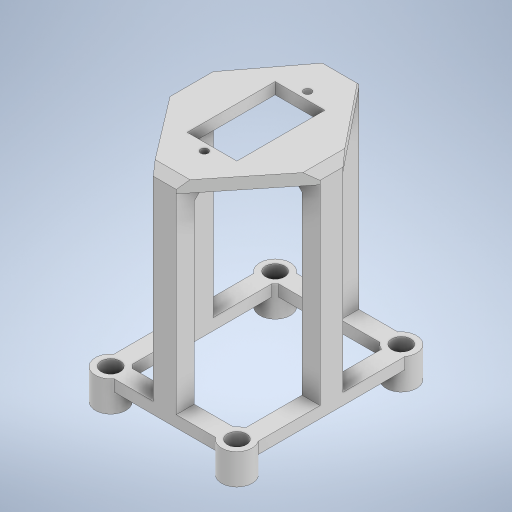
# Autodesk Inventor part: ServoMount
Saved by Autodesk Inventor 2024.2 (Build 282272000, 272)
## iProperties
Created: 2024-04-02
Part Number: ServoMount
Material: Generic
Document SubType Name: Modeling
Designer: ringl
Density: 1 g/cm^3
Appearance: Default
Author: ringl
Autodesk Inventor part; units mm, degrees
ref_plane "YZ Plane" through (0, 0, 0) normal (1, 0, 0) x (0, 1, 0)
ref_plane "XZ Plane" through (0, 0, 0) normal (0, 1, 0) x (-1, 0, 0)
ref_plane "XY Plane" through (0, 0, 0) normal (0, 0, 1) x (1, 0, 0)
sketch "Sketch1" plane through (0, 0, 0) normal (0, 1, 0) x (-1, 0, 0)
  circle A0 centre (0, 0) radius 2.5
  circle A1 centre (0, -43) radius 2.5
  circle A2 centre (-33, 0) radius 2.5
  circle A3 centre (-33, -43) radius 2.5
  line L0 (-3.2369, 2.35) -> (-29.7631, 2.35)
  line L1 (-29.7631, -2.35) -> (-3.2369, -2.35)
  line L2 (-2.35, -3.2369) -> (-2.35, -39.7631)
  line L3 (-3.2369, -40.65) -> (-29.7631, -40.65)
  line L4 (-31.5369, -39.2772) -> (-31.5369, -3.7228)
  line L5 (-36.2369, -2.35) -> (-36.2369, -40.65)
  line L6 (-3.2369, -45.35) -> (-29.7631, -45.35)
  arc A4 (-29.7631, -40.65) -> (-31.5369, -39.2772) centre (-33, -43) ccw
  arc A5 (-36.2369, -40.65) -> (-29.7631, -45.35) centre (-33, -43) ccw
  line L7 (2.35, -3.2369) -> (2.35, -39.7631)
  arc A6 (-3.2369, -45.35) -> (2.35, -39.7631) centre (0, -43) ccw
  arc A7 (-2.35, -39.7631) -> (-3.2369, -40.65) centre (0, -43) ccw
  arc A8 (2.35, -3.2369) -> (-3.2369, 2.35) centre (0, 0) ccw
  arc A9 (-3.2369, -2.35) -> (-2.35, -3.2369) centre (0, 0) ccw
  arc A10 (-29.7631, 2.35) -> (-36.2369, -2.35) centre (-33, 0) ccw
  arc A11 (-31.5369, -3.7228) -> (-29.7631, -2.35) centre (-33, 0) ccw
  point P0 (-16.5, 2.35)
  dimension "d0" = 5
  dimension "d1" = 5
  dimension "d2" = 5
  dimension "d3" = 5
  dimension "d8" = 4
  dimension "d9" = 4
  dimension "d10" = 4
  dimension "d11" = 4
  dimension "d12" = 4
  dimension "d13" = 4
  dimension "d18" = 43
  dimension "d23" = 33
  dimension "d24" = 4.7
  dimension "d25" = 4.7
  dimension "d26" = 4.7
  dimension "d27" = 4.7
  dimension "d28" = 2.35
  dimension "d29" = 2.35
  dimension "d30" = 4
  dimension "d31" = 2.35
  constraints: 16 end point, 16 point on circle, 12 centre point, 5 coincident, 3 perpendicular, 2 horizontal, 2 horizontal alignment, 2 point on line, 2 vertical alignment, 1 midpoint, 1 parallel, 1 vertical
  measures "d0" diameter of A0
  measures "d1" diameter of A1
  measures "d2" diameter of A2
  measures "d3" diameter of A3
  measures "d8" radius of A10
  measures "d9" radius of A11
  measures "d10" radius of A8
  measures "d11" radius of A9
  measures "d12" radius of A7
  measures "d13" radius of A6
  measures "d18" distance of A1.centre point (0, 0)
  measures "d23" distance of A2.centre point (0, 0)
  measures "d24" distance between parallel lines of L7 L2
  measures "d25" distance between parallel lines of L6 L3
  measures "d26" distance between parallel lines of L5 L4
  measures "d27" distance from line of point (-16.5, 2.35) L1
  measures "d28" distance from line of A2.centre L1
  measures "d29" distance from line of L3 A3.centre
  measures "d30" radius of A4
  measures "d31" distance from line of point (0, 0) L2
extrude "Extrusion1" add sketch "Sketch1" along normal blind 3
sketch "Sketch2" plane through (0, 0, 0) normal (0, -1, 0) x (1, 0, 0)
  circle A0 centre (0, 0) radius 2.5
  circle A1 centre (0, 0) radius 4
  arc A2 (36.2369, -2.35) -> (29.7631, 2.35) centre (33, 0) ccw projected
  circle A3 centre (33, 0) radius 2.5
  circle A4 centre (33, 0) radius 4
  arc A5 (-2.35, -39.7631) -> (3.2369, -45.35) centre (0, -43) ccw projected
  circle A6 centre (0, -43) radius 2.5
  line L0 (29.7631, -45.35) -> (3.2369, -45.35) projected
  circle A7 centre (0, -43) radius 4
  circle A8 centre (33, -43) radius 2.5
  circle A9 centre (33, -43) radius 4
  point P0 (-2.35, -39.7631)
  point P1 (29.7631, 2.35)
  point P2 (36.2369, -2.35)
  dimension "d34" = 5
  dimension "d35" = 8
  dimension "d37" = 8
  dimension "d38" = 5
  dimension "d39" = 5
  dimension "d40" = 5
  constraints: 7 centre point, 7 coincident, 1 concentric, 1 horizontal alignment, 1 vertical alignment, 3 other
  measures "d34" diameter of A0
  measures "d35" diameter of A1
  measures "d37" diameter of A9
  measures "d38" diameter of A8
  measures "d39" diameter of A6
  measures "d40" diameter of A3
extrude "Extrusion2" add sketch "Sketch2" along normal blind 5
sketch "Sketch3" plane through (0, 3, 0) normal (0, 1, 0) x (1, 0, 0)
  line L0 (3.2369, -2.35) -> (29.7631, -2.35) projected
  line L1 (29.7631, 2.35) -> (3.2369, 2.35) projected
  line L2 (13.5, -2.35) -> (19.5, -2.35)
  line L3 (19.5, -2.35) -> (19.5, 2.35)
  line L4 (19.5, 2.35) -> (13.5, 2.35)
  line L5 (13.5, 2.35) -> (13.5, -2.35)
  line L6 (31.5369, 39.2772) -> (31.5369, 3.7228) projected
  line L7 (36.2369, 2.35) -> (36.2369, 40.65) projected
  line L8 (31.5369, 18.5) -> (36.2369, 18.5)
  line L9 (36.2369, 18.5) -> (36.2369, 24.5)
  line L10 (36.2369, 24.5) -> (31.5369, 24.5)
  line L11 (31.5369, 24.5) -> (31.5369, 18.5)
  line L12 (3.2369, 40.65) -> (29.7631, 40.65) projected
  line L13 (29.7631, 45.35) -> (3.2369, 45.35) projected
  line L14 (19.5, 40.65) -> (13.5, 40.65)
  line L15 (13.5, 40.65) -> (13.5, 45.35)
  line L16 (13.5, 45.35) -> (19.5, 45.35)
  line L17 (19.5, 45.35) -> (19.5, 40.65)
  line L18 (2.35, 3.2369) -> (2.35, 39.7631) projected
  line L19 (-2.35, 39.7631) -> (-2.35, 3.2369) projected
  line L20 (2.35, 24.5) -> (-2.35, 24.5)
  line L21 (-2.35, 24.5) -> (-2.35, 18.5)
  line L22 (-2.35, 18.5) -> (2.35, 18.5)
  line L23 (2.35, 18.5) -> (2.35, 24.5)
  point P0 (0, 0)
  point P1 (13.5, 43)
  point P2 (19.5, 43)
  point P3 (-2.35, 24.5)
  dimension "d43" = 6
  dimension "d44" = 6
  dimension "d45" = 6
  dimension "d46" = 6
  dimension "d47" = 18.5
  dimension "d48" = 18.5
  dimension "d49" = 13.5
  dimension "d50" = 13.5
  constraints: 32 end point, 8 parallel, 8 point on line, 4 horizontal, 4 perpendicular, 2 midpoint
  measures "d43" distance between parallel lines of L5 L3
  measures "d44" distance between parallel lines of L10 L8
  measures "d45" distance of point (13.5, 43) point (19.5, 43)
  measures "d46" distance between parallel lines of L22 L20
  measures "d47" distance from line of L22 point (0, 0)
  measures "d48" distance from line of point (0, 0) L8
  measures "d49" distance from line of point (0, 0) L5
  measures "d50" distance from line of point (0, 0) L15
extrude "Extrusion3" add sketch "Sketch3" along normal blind 50
sketch "Sketch4" plane through (0, 53, 0) normal (0, 1, 0) x (1, 0, 0)
  line L0 (-2.35, 18.5) -> (-2.35, 24.5)
  line L1 (13.5, -2.35) -> (19.5, -2.35) projected
  line L2 (13.5, -2.35) -> (19.5, -2.35)
  line L3 (19.5, 45.35) -> (13.5, 45.35) projected
  line L4 (13.5, 45.35) -> (19.5, 45.35)
  line L5 (36.2369, 24.5) -> (31.5369, 24.5) projected
  line L6 (36.2369, 18.5) -> (36.2369, 24.5) projected
  line L7 (36.2369, 24.5) -> (36.2369, 18.5)
  line L8 (13.5, -2.35) -> (-2.35, 18.5)
  line L9 (-2.35, 24.5) -> (13.5, 45.35)
  line L10 (19.5, 45.35) -> (36.2369, 24.5)
  line L11 (36.2369, 18.5) -> (19.5, -2.35)
  line L12 (10, 10) -> (23, 10)
  line L13 (10, 10) -> (10, 33)
  line L14 (10, 33) -> (23, 33)
  line L15 (23, 10) -> (23, 33)
  point P0 (0, 0)
  dimension "d53" = 23
  dimension "d54" = 13
  dimension "d68" = 10
  dimension "d69" = 23
  dimension "d70" = 10
  constraints: 24 end point, 3 collinear, 2 horizontal, 1 vertical
  measures "d53" distance of L13.end L12.start
  measures "d54" distance of L14.end L13.end
  measures "d68" distance from line of point (0, 0) L13
  measures "d69" distance from line of point (0, 0) L15
  measures "d70" distance from line of point (0, 0) L12
extrude "Extrusion4" add sketch "Sketch4" along normal blind 3
sketch "Sketch5" plane through (0, 56, 0) normal (0, 1, 0) x (1, 0, 0)
  circle A0 centre (16.5, 35) radius 1
  circle A1 centre (16.5, 8) radius 1
  line L0 (10, 10) -> (10, 33) projected
  line L1 (23, 10) -> (10, 10) projected
  line L2 (10, 33) -> (23, 33) projected
  point P0 (0, 0)
  dimension "d73" = 2
  dimension "d74" = 2
  dimension "d75" = 6.5
  dimension "d76" = 6.5
  dimension "d77" = 2
  dimension "d78" = 2
  constraints: 2 centre point
  measures "d73" diameter of A0
  measures "d74" diameter of A1
  measures "d75" distance from line of L0 A1.centre
  measures "d76" distance from line of L0 A0.centre
  measures "d77" distance from line of L1 A1.centre
  measures "d78" distance from line of L2 A0.centre
extrude "Extrusion5" cut sketch "Sketch5" against normal blind 3
chamfer "Chamfer1" distance 4 angle 45 4 edges at (16.5, 53, -40.65) (31.5369, 53, -21.5) (16.5, 53, -2.35) (2.35, 53, -21.5)
chamfer "Chamfer2" distance 2 angle 45 4 edges at (16.5, 56, 2.35) (-2.35, 56, -21.5) (16.5, 56, -45.35) (36.2369, 56, -21.5)
body "Solid1"
